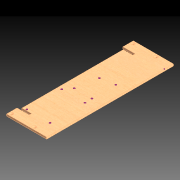
# Autodesk Inventor part: KB33-046-004-002 - Передняя пластина
Saved by Autodesk Inventor 2020 (Build 240168000, 168)
## iProperties
Created: 2021-06-25
Part Number: KB33-046-004-002 - Передняя пластина
Material: Дерево (вишня)
Document SubType Name: Modeling
Designer: Петров Иван
Mass: 51.2232 g
Surface Area: 443.017 cm^2
Volume: 81.3067 cm^3
Density: 0.63 g/cm^3
Appearance: Вишневое дерево — натуральный — со слабым глянцем
Author: Петров Иван
Autodesk Inventor part; units mm, degrees
ref_plane "YZ Plane" through (0, 0, 0) normal (1, 0, 0) x (0, 1, 0)
ref_plane "XZ Plane" through (0, 0, 0) normal (0, 1, 0) x (-1, 0, 0)
ref_plane "XY Plane" through (0, 0, 0) normal (0, 0, 1) x (1, 0, 0)
sketch "Эскиз1" plane through (0, 0, 0) normal (0, 1, 0) x (-1, 0, 0)
  line L0 (-2.6795, -19) -> (83.0251, -19)
  line L1 (-2.6795, 244) -> (83.0251, 244)
  circle A0 centre (30.7479, 238.5) radius 1.85
  circle A1 centre (78.7479, 238.5) radius 1.85
  circle A2 centre (78.7479, -13.5) radius 1.85
  circle A3 centre (30.7479, -13.5) radius 1.85
  line L2 (83.0251, 244) -> (-2.6795, 244)
  line L3 (-2.6795, 244) -> (-2.6795, -19)
  line L4 (-2.6795, -19) -> (83.0251, -19)
  line L5 (83.0251, -19) -> (83.0251, 244)
  point P0 (0, 0)
  point P1 (83.0251, -19)
  point P2 (-2.6795, 244)
  dimension "d7" = 5.5
  dimension "d8" = 5.5
  dimension "d9" = 4.2772
  dimension "d10" = 48
  dimension "d11" = 263
  dimension "d12" = 5.5
  dimension "d13" = 5.5
  dimension "d14" = 4.2772
  dimension "d15" = 48
  constraints: 12 end point, 4 centre point, 2 parallel, 1 horizontal, 1 perpendicular
  measures "d7" distance from line of L0 A3.centre
  measures "d8" distance from line of L0 A2.centre
  measures "d9" distance from line of L5 A2.centre
  measures "d10" distance of A2.centre A3.centre
  measures "d11" distance of L2.end L0.start
  measures "d12" distance from line of L1 A0.centre
  measures "d13" distance from line of L1 A1.centre
  measures "d14" distance from line of L5 A1.centre
  measures "d15" distance of A1.centre A0.centre
extrude "Выдавливание1" add sketch "Эскиз1" along normal blind 4
thicken "Толщина1" operation add thickness 2.671 both sides no extend neighbours yes toward (-1, 0, 0) faces at (2.6795, 1.3333, 156.3333)
chamfer "Фаска1" distance 2 angle 45 4 edges at (-76.8979, 4, 238.5) (-28.8979, 4, 238.5) (-28.8979, 4, -13.5) (-76.8979, 4, -13.5)
sketch "Эскиз2" plane through (-1.399, 4, 60) normal (0, 1, 0) x (1, 0, 0)
  line L0 (-76.2625, -157.5) -> (-76.2625, 52.5)
  line L1 (-76.2625, 52.5) -> (-56.2625, 52.5)
  line L2 (-56.2625, -157.5) -> (-76.2625, -157.5)
  line L3 (-56.2625, 57.5) -> (-76.2625, 57.5)
  line L4 (-76.2625, 57.5) -> (-81.2625, 57.5)
  line L5 (-81.2625, 57.5) -> (-81.2625, -162.5)
  line L6 (-81.2625, -162.5) -> (-76.2625, -162.5)
  line L7 (-76.2625, -162.5) -> (-56.2625, -162.5)
  line L8 (-56.2625, -162.5) -> (-56.2625, -157.5)
  line L9 (-56.2625, 52.5) -> (-56.2625, 57.5)
  line L10 (1.4075, -184) -> (1.4075, 79) projected
  point P0 (0, 0)
  dimension "d21" = 57.67
  dimension "d22" = 25
  dimension "d23" = 5
  constraints: 20 end point
  measures "d21" distance between parallel lines of L10 L8
  measures "d22" distance between parallel lines of L5 L8
  measures "d23" distance between parallel lines of L5 L0
extrude "Выдавливание2" cut sketch "Эскиз2" against normal blind 10
thicken "Толщина2" operation add thickness 2 both sides no extend neighbours yes toward (-1, 0, 0) faces at (-82.6615, 2.6667, 75.8333)
sketch "Эскиз3" plane through (0, 4, 0) normal (0, 1, 0) x (1, 0, 0)
  circle A0 centre (-51.7551, -83.34) radius 1.5 projected
  circle A1 centre (-22.5451, -78.26) radius 1.5 projected
  circle A2 centre (-22.5451, -127.79) radius 1.5 projected
  circle A3 centre (-59.3751, -127.79) radius 1.5 projected
  circle A4 centre (-22.2251, -142.53) radius 1.5 projected
  circle A5 centre (-70.4851, -142.53) radius 1.5 projected
  circle A6 centre (-22.2251, -214.92) radius 1.5 projected
  circle A7 centre (-70.4851, -214.92) radius 1.5 projected
  point P0 (0, 0)
extrude "Выдавливание3" cut sketch "Эскиз3" against normal blind 10
